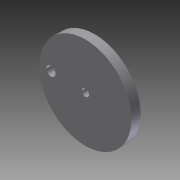
# Autodesk Inventor part: tiltBoxGearSpacerBlock
Saved by Autodesk Inventor 2012 (Build 160160000, 160)
## iProperties
Created: 2014-06-13
Part Number: tiltBoxGearSpacerBlock
Material: Default
Document SubType Name: Modeling
Designer: Byron
Density: 1 g/cm^3
Author: Byron
Autodesk Inventor part; units mm, degrees
ref_plane "YZ Plane" through (0, 0, 0) normal (1, 0, 0) x (0, 1, 0)
ref_plane "XZ Plane" through (0, 0, 0) normal (0, 1, 0) x (-1, 0, 0)
ref_plane "XY Plane" through (0, 0, 0) normal (0, 0, 1) x (1, 0, 0)
sketch "Sketch1" plane through (0, 0, 0) normal (0, 0, 1) x (1, 0, 0)
  circle A0 centre (-21.3276, -21.2251) radius 2.5 projected
  circle A1 centre (-45.0763, -20.2868) radius 3.175 projected
  circle A2 centre (-21.3276, -21.2251) radius 31.75
  point P0 (0, 0)
  dimension "d0" = 63.5
  constraints: 1 centre point, 1 coincident
  measures "d0" diameter of A2
extrude "Extrusion1" add sketch "Sketch1" along normal blind 6.35
body "Solid1"
